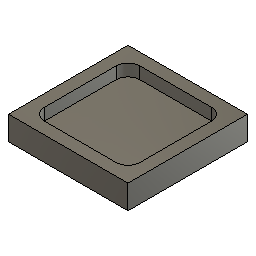
sample (Autodesk Fusion 360 design; units mm, degrees)
Autodesk Fusion 360 part; units mm, degrees
sketch "Sketch1" plane through (0, 0, 0) normal (0, 1, 0) x (1, 0, 0)
  line L0 (0, 0) -> (100, 0)
  line L1 (100, 0) -> (100, 100)
  line L2 (100, 100) -> (0, 100)
  line L3 (0, 100) -> (0, 0)
  dimension "d1" = 100
  dimension "d2" = 100
  constraint horizontal L0
  constraint vertical L1
  constraint horizontal L2
  constraint vertical L3
  constraint coincident L0.start L3.end
  measures "d1" distance of L0.end L1.end
  measures "d2" distance of L1.end L2.end
extrude "Extrude1" add sketch "Sketch1" along normal blind 20
sketch "Sketch2" plane through (0, 20, 0) normal (0, 1, 0) x (-1, 0, 0)
  line L0 (0, -100) -> (0, 0)
  line L1 (0, 0) -> (-100, 0)
  line L2 (-100, 0) -> (-100, -100)
  line L3 (-100, -100) -> (0, -100)
  line L4 (-10, -10) -> (-90, -10)
  line L5 (-90, -10) -> (-90, -90)
  line L6 (-90, -90) -> (-10, -90)
  line L7 (-10, -90) -> (-10, -10)
  dimension "d5" = 80
  dimension "d6" = 80
  dimension "d7" = 10
  dimension "d8" = 10
  constraint horizontal L4
  constraint vertical L5
  constraint horizontal L6
  constraint vertical L7
  measures "d5" distance of L4.end L5.end
  measures "d6" distance of L5.end L6.end
  measures "d7" distance of L0 L4.start
  measures "d8" vertical distance of L0.end L4.start
extrude "Extrude2" cut sketch "Sketch2" against normal blind 10 contours L4 L5 L6 L7
fillet "Fillet1" radius 10 4 edges at (10, 15, -10) (10, 15, -90) (90, 15, -90) (90, 15, -10)
